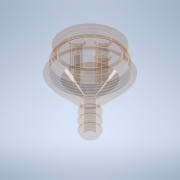
# Autodesk Inventor part: Bottom
Saved by Autodesk Inventor 2021 (Build 250183000, 183)
## iProperties
Created: 2021-08-11
Part Number: Bottom
Material: Polycarbonate, Smoke
Document SubType Name: Modeling
Designer: incep
Density: 1.2 g/cm^3
Appearance: Polycarbonate - Smoked
Author: incep
## iProperties of the stored document _3DPrint.ipt
Created: 2021-08-11
Part Number: _3DPrint
Material: Generic
Document SubType Name: Modeling
Designer: incep
Density: 1 g/cm^3
Appearance: Default
Author: incep
Autodesk Inventor part; units mm, degrees
ref_plane "YZ Plane" through (0, 0, 0) normal (1, 0, 0) x (0, 1, 0)
ref_plane "XZ Plane" through (0, 0, 0) normal (0, 1, 0) x (-1, 0, 0)
ref_plane "XY Plane" through (0, 0, 0) normal (0, 0, 1) x (1, 0, 0)
sketch "Bottom Sketch" plane through (0, 0, 0) normal (0, 0, 1) x (1, 0, 0)
  line L0 (-17, 0) -> (17, 0) construction
  line L1 (17, 0) -> (17, -8) construction
  line L2 (17, -8) -> (-17, -8) construction
  line L3 (-17, -8) -> (-17, 0) construction
  line L4 (-14.5, 0) -> (14.5, 0) construction
  line L5 (14.5, 0) -> (14.5, -8) construction
  line L6 (14.5, -8) -> (-14.5, -8) construction
  line L7 (-14.5, -8) -> (-14.5, 0) construction
  line L8 (17, -8) -> (17, -5.8)
  line L9 (17, -5.8) -> (14.5, -5.8)
  line L10 (14.5, -5.8) -> (14.5, -2)
  line L11 (14.5, -2) -> (17, -2)
  line L12 (17, -2) -> (17, 0)
  line L13 (17, -8) -> (18.1014, -8)
  line L14 (-6.5, 0) -> (6.5, 0) construction
  line L15 (6.5, 0) -> (6.5, -30) construction
  line L16 (6.5, -30) -> (-6.5, -30) construction
  line L17 (-6.5, -30) -> (-6.5, 0) construction
  line L18 (18.1014, -8) -> (18.1014, -15)
  line L19 (17, 0) -> (0, 0)
  line L20 (-4.5, -30) -> (4.5, -30) construction
  line L21 (4.5, -48) -> (-4.5, -48) construction
  line L22 (-4.5, -48) -> (-4.5, -30) construction
  line L23 (6.5, -30) -> (4.5, -30)
  line L24 (4.5, -48) -> (2.75, -48)
  line L25 (2.75, -48) -> (2.75, -28.3188)
  line L26 (0, 0) -> (0, -18)
  line L27 (0, -18) -> (13.0688, -18)
  line L28 (13.0688, -18) -> (2.75, -28.3188)
  line L29 (-1.7435, -30) -> (1.7435, -30) construction
  line L30 (1.7435, -30) -> (1.7435, -48) construction
  line L31 (1.7435, -48) -> (-1.7435, -48) construction
  line L32 (-1.7435, -48) -> (-1.7435, -30) construction
  line L33 (4.5, -45) -> (5.5, -45) construction
  line L34 (5.5, -45) -> (5.5, -48) construction
  line L35 (5.5, -48) -> (4.5, -48) construction
  line L36 (4.5, -48) -> (4.5, -45) construction
  line L37 (4.5, -40) -> (5.5, -40) construction
  line L38 (5.5, -40) -> (5.5, -43) construction
  line L39 (5.5, -43) -> (4.5, -43) construction
  line L40 (4.5, -43) -> (4.5, -40) construction
  line L41 (4.5, -35) -> (5.5, -35) construction
  line L42 (5.5, -35) -> (5.5, -38) construction
  line L43 (5.5, -38) -> (4.5, -38) construction
  line L44 (4.5, -38) -> (4.5, -35) construction
  line L45 (4.5, -48) -> (5.5, -46)
  line L46 (5.5, -45) -> (5.5, -46)
  line L47 (5.5, -45) -> (4.5, -45)
  line L48 (4.5, -43) -> (5.5, -41)
  line L49 (5.5, -41) -> (5.5, -40)
  line L50 (5.5, -40) -> (4.5, -40)
  line L51 (4.5, -38) -> (5.5, -36)
  line L52 (5.5, -36) -> (5.5, -35)
  line L53 (5.5, -35) -> (4.5, -35)
  line L54 (4.5, -30) -> (4.5, -35)
  line L55 (4.5, -30) -> (4.5, -40) construction
  line L56 (4.5, -43) -> (4.5, -45) construction
  line L57 (4.5, -38) -> (4.5, -40)
  line L58 (4.5, -43) -> (4.5, -45)
  line L59 (-22.5, 0) -> (22.5, 0) construction
  line L60 (22.5, 0) -> (22.5, -15) construction
  line L61 (22.5, -15) -> (-22.5, -15) construction
  line L62 (-22.5, -15) -> (-22.5, 0) construction
  line L63 (-21.5, 0) -> (21.5, 0) construction
  line L64 (21.5, 0) -> (21.5, -15) construction
  line L65 (21.5, -15) -> (-21.5, -15) construction
  line L66 (-21.5, -15) -> (-21.5, 0) construction
  line L67 (22.5, 0) -> (21.7499, -11.251) construction
  line L68 (18.8432, -17.6568) -> (6.5, -30)
  arc A0 (18.8432, -17.6568) -> (20.7451, -15) centre (11.7721, -10.5858) ccw
  line L69 (18.1014, -15) -> (20.7451, -15)
  point P0 (0, -8)
  point P1 (0, -30)
  point P2 (0, -30)
  point P3 (0, -30)
  point P4 (0, -48)
  point P5 (0, -48)
  dimension "d0" = 8
  dimension "d1" = 8
  dimension "d2" = 34
  dimension "d3" = 29
  dimension "d4" = 2
  dimension "d5" = 3.8
  dimension "d6" = 30
  dimension "d7" = 13
  dimension "d8" = 9
  dimension "d9" = 18
  dimension "d10" = 1.75
  dimension "d11" = 18
  dimension "d16" = 1
  dimension "d18" = 3
  dimension "d19" = 1
  dimension "d20" = 3
  dimension "d21" = 2
  dimension "d22" = 1
  dimension "d23" = 3
  dimension "d24" = 2
  dimension "d25" = 15
  dimension "d26" = 1
  dimension "d27" = 1
  dimension "d28" = 1
  dimension "d29" = 15
  dimension "d30" = 45
  dimension "d31" = 15
  dimension "d32" = 43
  dimension "d33" = 10
  constraints: 140 end point, 22 parallel, 16 perpendicular, 14 coincident, 14 collinear, 12 horizontal, 12 point on line, 11 midpoint, 2 point on circle, 2 tangent, 2 vertical alignment, 1 centre point, 1 vertical
  measures "d0" distance of L1.start L8.start
  measures "d1" distance of L5.start L5.end
  measures "d2" distance of L8.start L2.end
  measures "d3" distance of L5.end L6.end
  measures "d4" distance of L11.end L1.start
  measures "d5" distance of L9.end L10.end
  measures "d6" distance of L15.end L15.start
  measures "d7" distance of L15.end L17.start
  measures "d8" distance of L24.start L22.start
  measures "d9" distance of L20.end L24.start
  measures "d10" distance of L24.start L25.start
  measures "d11" distance of L19.end L26.end
  measures "d16" distance of L34.end L24.start
  measures "d18" distance of L33.end L34.end
  measures "d19" distance of L38.end L39.end
  measures "d20" distance of L37.end L38.end
  measures "d21" distance of L33.start L39.end
  measures "d22" distance of L42.end L43.end
  measures "d23" distance of L41.end L42.end
  measures "d24" distance of L37.start L43.end
  measures "d25" vertical distance of L18.end point (0, 0)
  measures "d26" distance of L33.end L45.end
  measures "d27" distance of L48.end L37.end
  measures "d28" distance of L51.end L41.end
  measures "d29" distance of L61.end L59.start
  measures "d30" distance of L60.end L61.end
  measures "d31" distance of L65.end L63.start
  measures "d32" distance of L63.start L63.end
  measures "d33" radius of A0
revolve "Bottom" add sketch "Bottom Sketch" angle 360 about axis through (0, 0, 0) along (0, -1, 0)
thread "Thread2" size "M38x1.5" class "6g" standard "ANSI Metric M Profile" full length
sketch "Sketch2" plane through (0, 0, 0) normal (0, 1, 0) x (1, 0, 0)
  circle A0 centre (8, 0) radius 2.65
  circle A1 centre (0, 8) radius 2.65
  circle A2 centre (-8, 0) radius 2.65
  circle A3 centre (0, -8) radius 1.5
  point P0 (0, 0)
  point P1 (0, 0)
  point P2 (0, 0)
  dimension "d37" = 8
  dimension "d38" = 5.3
  dimension "d41" = 180
  dimension "d43" = 8
  dimension "d44" = 3
  constraints: 4 centre point, 1 coincident, 6 other
  measures "d37" distance of A0.centre point (0, 0)
  measures "d38" diameter of A0
  measures "d43" distance of A3.centre point (0, 0)
  measures "d44" diameter of A3
extrude "Extrusion1" cut sketch "Sketch2" against normal blind 19
sketch "Sketch3" plane through (0, 0, 0) normal (0, 1, 0) x (1, 0, 0)
  circle A0 centre (8, 0) radius 4
  circle A1 centre (0, 8) radius 4
  circle A2 centre (-8, 0) radius 4
  point P0 (0, 0)
  point P1 (0, 0)
  point P2 (0, 0)
  dimension "d47" = 8
  dimension "d49" = 8
  dimension "d52" = 180
  constraints: 3 centre point, 1 coincident, 1 horizontal alignment, 6 other
  measures "d47" diameter of A0
  measures "d49" distance of A0.centre point (0, 0)
extrude "Extrusion2" cut sketch "Sketch3" against normal blind 2.36
sketch "Sketch4" plane through (0, 0, 0) normal (0, 1, 0) x (1, 0, 0)
  circle A0 centre (0, 8) radius 2.65 projected
  circle A1 centre (0, 5.35) radius 1.5
  circle A2 centre (8, 0) radius 2.65 projected
  circle A3 centre (8, -2.65) radius 1.5
  circle A4 centre (-8, 0) radius 2.65 projected
  circle A5 centre (-8, -2.65) radius 1.5
  point P0 (0, 0)
  dimension "d56" = 3
  dimension "d57" = 3
  dimension "d58" = 3
  constraints: 3 centre point, 3 vertical alignment, 3 other
  measures "d56" diameter of A1
  measures "d57" diameter of A3
  measures "d58" diameter of A5
extrude "Extrusion3" cut sketch "Sketch4" against normal blind 19 contours A1 A0 | A0 A1 | A3 A2 | A2 A3 | A5 A4 | A4 A5 picked at (0.0582, 5.8582) picked at (0.0506, 4.8642) picked at (8.0582, -2.1418) picked at (8.0506, -3.1358) picked at (-7.9418, -2.1418) picked at (-7.9494, -3.1358)
body "Solid2"
